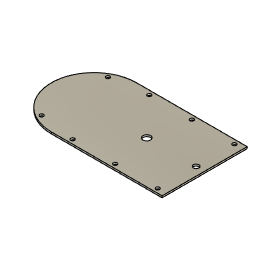
weight_lids v37 (Autodesk Fusion 360 design; units mm, degrees)
Autodesk Fusion 360 part; units mm, degrees
note: some values were not read from the file. Chosen so that the rebuilt part matches the saved one: which face or edge a step refers to; how an offset face is resized. Set by a fixed rule: which sketch regions a step uses.
sketch "Sketch1" plane through (0, 0, 0) normal (0, 0, 1) x (1, 0, 0)
  circle A0 centre (0, 0) radius 45.2465
  dimension "d1" = 90.493
  constraint coincident A0.centre origin
  measures "d1" diameter of A0
sketch "Sketch2" plane through (0, 0, 0) normal (0, 0, 1) x (1, 0, 0)
  circle A0 centre (0, 0) radius 50
  line L0 (0, 0) -> (300, 0)
  line L1 (0, 0) -> (-50, 0)
  circle A1 centre (300, 0) radius 50
  line L2 (300, 0) -> (350, 0)
  line L3 (300, 50) -> (0, 50)
  dimension "d4" = 100
  dimension "d5" = 300
  dimension "d6" = 100
  constraint coincident A0.centre L0.start
  constraint horizontal L0
  constraint coincident A0 L1.end
  constraint parallel L0 L1
  constraint coincident L0.end A1.centre
  constraint coincident A1 L2.end
  constraint parallel L0 L2
  constraint coincident A1 L3.start
  constraint coincident A0 L3.end
  constraint tangent A0 L3
  constraint parallel L0 L3
  measures "d4" diameter of A0
  measures "d5" distance of A0.centre L0.end
  measures "d6" diameter of A1
extrude "Extrude2" add sketch "Sketch2" along normal blind 2 contours A0 L0 L1 | A0 L0 A1 L3 | L0 A1 L2 picked at (-33.1637, 2.3719) picked at (266.8363, 2.3719) makes body 1
sketch "Sketch3" plane through (0, 0, 2) normal (0, 0, 1) x (-1, 0, 0)
  line L0 (50, 0) -> (-350, 0)
  arc A0 (-350, 0) -> (-300, -50) centre (-300, 0) ccw
  line L1 (-300, -50) -> (0, -50)
  arc A1 (0, -50) -> (50, 0) centre (0, 0) ccw
  circle A2 centre (-150, 0) radius 12.7
  dimension "d9" = 25.4
  constraint midpoint L0 A2.centre
  measures "d9" diameter of A2
extrude "Extrude3" cut sketch "Sketch3" against normal blind 30 contours L0 A2 picked at (-150.3164, -4.2215) bodies 1
sketch "Sketch4" plane through (0, 0, 2) normal (0, 0, 1) x (-1, 0, 0)
  arc A0 (-162.7, 0) -> (-137.3, 0) centre (-150, 0) ccw
  line L0 (-162.7, 0) -> (-350, 0)
  arc A1 (-350, 0) -> (-300, -50) centre (-300, 0) ccw
  line L1 (-300, -50) -> (0, -50)
  arc A2 (0, -50) -> (50, 0) centre (0, 0) ccw
  line L2 (50, 0) -> (-137.3, 0)
  circle A3 centre (0, 0) radius 45
  circle A4 centre (-300, 0) radius 45
  line L3 (0, 0) -> (0, -45)
  line L4 (0, -45) -> (-300, -45)
  line L5 (-45, 0) -> (22.5, -38.9711)
  line L6 (22.5, -38.9711) -> (22.5, 38.9711)
  line L7 (22.5, 38.9711) -> (-45, 0)
  line L8 (-255, 0) -> (-322.5, 38.9711)
  line L9 (-322.5, 38.9711) -> (-322.5, -38.9711)
  line L10 (-322.5, -38.9711) -> (-255, 0)
  line L11 (-75, -45) -> (-225, -45)
  line L12 (-225, -45) -> (-225, 0)
  line L13 (-225, 0) -> (-75, 0)
  line L14 (-75, 0) -> (-75, -45)
  line L15 (-175, 0) -> (-125, 0)
  line L16 (-125, 0) -> (-125, -45)
  line L17 (-125, -45) -> (-175, -45)
  line L18 (-175, -45) -> (-175, 0)
  line L19 (-75, 0) -> (-25, 0)
  line L20 (-25, 0) -> (-25, -45)
  line L21 (-25, -45) -> (-75, -45)
  line L22 (-75, -45) -> (-75, 0)
  line L23 (-225, 0) -> (-275, 0)
  line L24 (-275, 0) -> (-275, -45)
  line L25 (-275, -45) -> (-225, -45)
  line L26 (-225, -45) -> (-225, 0)
  point P0 (-300, 0)
  dimension "d12" = 90
  dimension "d13" = 90
  constraint concentric A2 A3
  constraint concentric A1 A4
  constraint coincident A2.centre A3.centre
  constraint coincident A3 L3.end
  constraint perpendicular L2 L3
  constraint coincident A4 L4.end
  constraint tangent A4 L4
  constraint coincident L2 L5.start
  constraint coincident A3 L5.start
  constraint coincident L0 L8.start
  constraint coincident A4 L8.start
  constraint coincident P0 A1.centre
  constraint horizontal L11
  constraint vertical L12
  constraint horizontal L13
  constraint vertical L14
  constraint coincident L0 L12.end
  constraint coincident L4 L11.start
  constraint horizontal L15
  constraint vertical L16
  constraint horizontal L17
  constraint vertical L18
  constraint coincident L4 L16.end
  constraint coincident L13 L15.start
  constraint horizontal L19
  constraint vertical L20
  constraint horizontal L21
  constraint vertical L22
  constraint coincident L4 L20.end
  constraint horizontal L23
  constraint vertical L24
  constraint horizontal L25
  constraint vertical L26
  constraint coincident L4 L24.end
  measures "d12" diameter of A3
  measures "d13" diameter of A4
hole "Hole1" at (-22.5, 38.9711, 2) at (25, 45, 2) at (75, 45, 2) at (125, 45, 2) at (175, 45, 2) at (225, 45, 2) at (275, 45, 2) at (322.5, 38.9711, 2) direction (0, 0, -1) diameter 3.529 depth 70 tip angle 180 bodies 1
thread "Thread1" "ISO Metric profile 4.0 M4x0.5 6H"
sketch "Sketch5" plane through (0, 0, 0) normal (0, 0, 1) x (1, 0, 0)
  circle A0 centre (0, 0) radius 50
  circle A1 centre (300, 0) radius 50
  circle A2 centre (150, 0) radius 12.7
  line L0 (0, -50) -> (300, -50)
  line L1 (50, 0) -> (137.3, 0)
  line L2 (162.7, 0) -> (250, 0)
  line L3 (-50, 0) -> (350, 0)
  dimension "d17" = 25.4
  constraint coincident A0.centre origin
  constraint coincident A0 L0.start
  constraint coincident A1 L0.end
  constraint tangent A1 L0
  constraint horizontal L0
  constraint coincident A0 L1.start
  constraint coincident A2 L1.end
  constraint parallel L0 L1
  constraint coincident A2 L2.start
  constraint coincident A1 L2.end
  constraint parallel L1 L2
  constraint coincident A0 L3.start
  constraint coincident A1 L3.end
  constraint horizontal L3
  measures "d17" diameter of A2
extrude "Extrude4" add sketch "Sketch5" along normal blind 2 contours A0 A1 A2 L0 L1 L2 L3 | A0 L3 | A1 L3 picked at (-6.9236, -15.1605) picked at (285.9791, -9.0107) bodies 1
sketch "Sketch6" plane through (0, 0, 2) normal (0, 0, 1) x (-1, 0, 0)
  circle A0 centre (-150, 0) radius 12.7
  circle A1 centre (-275, -45) radius 1.7644
  circle A2 centre (-175, -45) radius 1.7644
  circle A3 centre (-75, -45) radius 1.7644
  circle A4 centre (22.5, -38.9711) radius 1.7644
  circle A5 centre (-25, -45) radius 1.7644
  circle A6 centre (-125, -45) radius 1.7644
  circle A7 centre (-225, -45) radius 1.7644
  circle A8 centre (-322.5, -38.9711) radius 1.7644
  arc A9 (0, -50) -> (0, 50) centre (0, 0) ccw
  line L0 (0, 50) -> (-300, 50)
  arc A10 (-300, 50) -> (-300, -50) centre (-300, 0) ccw
  line L1 (-300, -50) -> (0, -50)
  line L2 (22.5, -38.9711) -> (22.5, 38.9711)
  line L3 (22.5, 38.9711) -> (-45, 0)
  line L4 (-45, 0) -> (22.5, -38.9711)
  line L5 (-322.5, -38.9711) -> (-255, 0)
  line L6 (-255, 0) -> (-322.5, 38.9711)
  line L7 (-322.5, 38.9711) -> (-322.5, -38.9711)
  line L8 (-25, -45) -> (-25, 50)
  line L9 (-25, 50) -> (-25, 45)
  line L10 (-25, -45) -> (-275, -45)
  line L11 (-275, -45) -> (-275, 45)
  line L12 (-275, 45) -> (-25, 45)
  line L13 (-25, 45) -> (-25, -45)
  line L14 (-25, -45) -> (-75, -45)
  line L15 (-75, -45) -> (-75, 45)
  line L16 (-75, 45) -> (-25, 45)
  line L17 (-25, 45) -> (-25, -45)
  line L18 (-75, -45) -> (-125, -45)
  line L19 (-125, -45) -> (-125, 45)
  line L20 (-125, 45) -> (-75, 45)
  line L21 (-75, 45) -> (-75, -45)
  line L22 (-175, -45) -> (-125, -45)
  line L23 (-125, -45) -> (-125, 45)
  line L24 (-125, 45) -> (-175, 45)
  line L25 (-175, 45) -> (-175, -45)
  line L26 (-225, -45) -> (-175, -45)
  line L27 (-175, -45) -> (-175, 45)
  line L28 (-175, 45) -> (-225, 45)
  line L29 (-225, 45) -> (-225, -45)
  point P0 (-300, 0)
  dimension "d20" = 5
  dimension "d21" = 250
  dimension "d22" = 90
  constraint coincident A4.centre L2.start
  constraint coincident A9.centre origin
  constraint coincident A8.centre L5.start
  constraint coincident P0 A10.centre
  constraint coincident A5.centre L8.start
  constraint coincident L0 L8.end
  constraint perpendicular L0 L8
  constraint perpendicular L0 L9
  constraint horizontal L10
  constraint vertical L11
  constraint horizontal L12
  constraint vertical L13
  constraint horizontal L14
  constraint vertical L15
  constraint horizontal L16
  constraint vertical L17
  constraint coincident L12 L15.end
  constraint horizontal L18
  constraint vertical L19
  constraint horizontal L20
  constraint vertical L21
  constraint coincident L12 L19.end
  constraint horizontal L22
  constraint vertical L23
  constraint horizontal L24
  constraint vertical L25
  constraint coincident A2.centre L22.start
  constraint horizontal L26
  constraint vertical L27
  constraint horizontal L28
  constraint vertical L29
  constraint coincident A7.centre L26.start
  measures "d20" distance of L8.end L9.end
  measures "d21" distance of A5.centre A1.centre
  measures "d22" distance of A5.centre L9.end
hole "Hole2" at (-22.5, -38.9711, 2) at (25, -45, 2) at (75, -45, 2) at (125, -45, 2) at (175, -45, 2) at (225, -45, 2) at (275, -45, 2) at (322.5, -38.9711, 2) direction (0, 0, -1) diameter 3.529 depth 70 tip angle 180 bodies 1
thread "Thread2" "ISO Metric profile 4.0 M4x0.5 6H"
sketch "Sketch7" plane through (0, 0, 2) normal (0, 0, 1) x (-1, 0, 0)
  circle A0 centre (-275, 45) radius 1.7644
  circle A1 centre (-175, 45) radius 1.7644
  circle A2 centre (-75, 45) radius 1.7644
  circle A3 centre (22.5, 38.9711) radius 1.7644
  circle A4 centre (-25, 45) radius 1.7644
  circle A5 centre (-125, 45) radius 1.7644
  circle A6 centre (-225, 45) radius 1.7644
  circle A7 centre (-322.5, 38.9711) radius 1.7644
  circle A8 centre (-150, 0) radius 12.7
  circle A9 centre (-275, -45) radius 1.7644
  circle A10 centre (-175, -45) radius 1.7644
  circle A11 centre (-75, -45) radius 1.7644
  circle A12 centre (22.5, -38.9711) radius 1.7644
  circle A13 centre (-25, -45) radius 1.7644
  circle A14 centre (-125, -45) radius 1.7644
  circle A15 centre (-225, -45) radius 1.7644
  circle A16 centre (-322.5, -38.9711) radius 1.7644
  arc A17 (0, -50) -> (0, 50) centre (0, 0) ccw
  line L0 (0, 50) -> (-300, 50)
  arc A18 (-300, 50) -> (-300, -50) centre (-300, 0) ccw
  line L1 (-300, -50) -> (0, -50)
  line L2 (-150, 0) -> (-130, 0)
  line L3 (-130, 0) -> (-130, -20)
  line L4 (-130, -20) -> (-150, -20)
  line L5 (-150, -20) -> (-150, 0)
  line L6 (-130, -20) -> (-170, -20)
  line L7 (-170, -20) -> (-170, 20)
  line L8 (-170, 20) -> (-130, 20)
  line L9 (-130, 20) -> (-130, -20)
  dimension "d26" = 40
  dimension "d27" = 40
  constraint horizontal L2
  constraint vertical L3
  constraint horizontal L4
  constraint vertical L5
  constraint coincident A8.centre L2.start
  constraint horizontal L6
  constraint vertical L7
  constraint horizontal L8
  constraint vertical L9
  measures "d26" distance of L3.end L6.end
  measures "d27" distance of L3.end L8.end
hole "Hole3" at (130, 20, 2) at (130, -20, 2) at (170, -20, 2) at (170, 20, 2) direction (0, 0, -1) diameter 3.332 depth 70 tip angle 180 bodies 1
ref_plane "WorkPlane1" through (150, 0, 0) normal (1, 0, 0) x (0, 1, 0)
split "Split1" by plane through (150, 0, 0) normal (1, 0, 0) bodies 1 makes body 2 at (206.7848, -6.4118, 0)
sketch "Sketch8" plane through (0, 0, 2) normal (0, 0, 1) x (-1, 0, 0)
  line L0 (-150, -12.7) -> (-150, -50)
  line L1 (-150, -50) -> (0, -50)
  arc A0 (0, -50) -> (0, 50) centre (0, 0) ccw
  line L2 (0, 50) -> (-150, 50)
  line L3 (-150, 50) -> (-150, 12.7)
  arc A1 (-150, -12.7) -> (-150, 12.7) centre (-150, 0) ccw
  circle A2 centre (-130, -20) radius 1.666
  circle A3 centre (-130, 20) radius 1.666
  circle A4 centre (-75, 45) radius 1.7644
  circle A5 centre (22.5, 38.9711) radius 1.7644
  circle A6 centre (-25, 45) radius 1.7644
  circle A7 centre (-125, 45) radius 1.7644
  circle A8 centre (-75, -45) radius 1.7644
  circle A9 centre (22.5, -38.9711) radius 1.7644
  circle A10 centre (-25, -45) radius 1.7644
  circle A11 centre (-125, -45) radius 1.7644
  line L4 (-150, 0) -> (-62, 0)
  line L5 (-150, 0) -> (-238, 0)
  dimension "d32" = 88
  dimension "d33" = 88
  constraint coincident A1.centre L4.start
  constraint parallel L1 L4
  constraint parallel L4 L5
  measures "d32" distance of A1.centre L4.end
  measures "d33" distance of A1.centre L5.end
hole "Hole4" at (62, 0, 2) at (238, 0, 2) direction (0, 0, -1) diameter 6.78 depth 70 tip angle 180 bodies 1 2
thread "Thread4" "ISO Metric profile 8.0 M8x1 6H" major diameter 8.147 minor diameter 7.035 pitch 1 angle 60 resizes the face on face at (62.3375, -3.3732, 1.3333) on face at (238.6717, -3.3228, 1.3333) on bodies 1 2
sketch "Sketch9" plane through (0, 0, 2) normal (0, 0, 1) x (-1, 0, 0)
  circle A0 centre (-62, 0) radius 3.5175
  line L0 (-150, -12.7) -> (-150, -50)
  line L1 (-150, -50) -> (0, -50)
  arc A1 (0, -50) -> (0, 50) centre (0, 0) ccw
  line L2 (0, 50) -> (-150, 50)
  line L3 (-150, 50) -> (-150, 12.7)
  arc A2 (-150, -12.7) -> (-150, 12.7) centre (-150, 0) ccw
  circle A3 centre (-130, -20) radius 1.666
  circle A4 centre (-130, 20) radius 1.666
  circle A5 centre (-75, 45) radius 1.7644
  circle A6 centre (22.5, 38.9711) radius 1.7644
  circle A7 centre (-25, 45) radius 1.7644
  circle A8 centre (-125, 45) radius 1.7644
  circle A9 centre (-75, -45) radius 1.7644
  circle A10 centre (22.5, -38.9711) radius 1.7644
  circle A11 centre (-25, -45) radius 1.7644
  circle A12 centre (-125, -45) radius 1.7644
  circle A13 centre (-150, 0) radius 17.4
  dimension "d37" = 34.8
  constraint concentric A2 A13
  measures "d37" diameter of A13
extrude "Extrude5" cut sketch "Sketch9" against normal blind 10 contours L0 L3 A2 A13 | L0 L3 A2 A13 bodies 1 2
sketch "Sketch10" plane through (0, 0, 2) normal (0, 0, 1) x (-1, 0, 0)
  circle A0 centre (-125, -45) radius 1.7644
  circle A1 centre (-25, -45) radius 1.7644
  circle A2 centre (22.5, -38.9711) radius 1.7644
  circle A3 centre (-75, -45) radius 1.7644
  circle A4 centre (-125, 45) radius 1.7644
  circle A5 centre (-25, 45) radius 1.7644
  circle A6 centre (22.5, 38.9711) radius 1.7644
  circle A7 centre (-75, 45) radius 1.7644
  circle A8 centre (-130, 20) radius 1.666
  circle A9 centre (-130, -20) radius 1.666
  arc A10 (-150, -17.4) -> (-150, 17.4) centre (-150, 0) ccw
  line L0 (-150, -17.4) -> (-150, -50)
  line L1 (-150, -50) -> (0, -50)
  arc A11 (0, -50) -> (0, 50) centre (0, 0) ccw
  line L2 (0, 50) -> (-150, 50)
  line L3 (-150, 50) -> (-150, 17.4)
  circle A12 centre (-62, 0) radius 3.5175
  circle A13 centre (-150, 0) radius 12.7
  circle A14 centre (-150, 0) radius 17.4
  line L4 (-150, -17.4) -> (-150, 17.4)
  dimension "d40" = 25.4
  constraint concentric A10 A13
  constraint concentric A13 A14
  constraint coincident A10.start L0.start
  constraint coincident A10.end L3.end
  measures "d40" diameter of A13
extrude "Extrude6" add sketch "Sketch10" against normal blind 2 contours A10 A13 A14 L4 bodies 1
sketch "Sketch11" plane through (0, 0, 2) normal (0, 0, 1) x (-1, 0, 0)
  circle A0 centre (-170, 20) radius 1.666
  circle A1 centre (-170, -20) radius 1.666
  circle A2 centre (-275, 45) radius 1.7644
  circle A3 centre (-175, 45) radius 1.7644
  circle A4 centre (-225, 45) radius 1.7644
  circle A5 centre (-322.5, 38.9711) radius 1.7644
  arc A6 (-150, 17.4) -> (-150, -17.4) centre (-150, 0) ccw
  line L0 (-150, 17.4) -> (-150, 50)
  line L1 (-150, 50) -> (-300, 50)
  arc A7 (-300, 50) -> (-300, -50) centre (-300, 0) ccw
  line L2 (-300, -50) -> (-150, -50)
  line L3 (-150, -50) -> (-150, -17.4)
  circle A8 centre (-275, -45) radius 1.7644
  circle A9 centre (-175, -45) radius 1.7644
  circle A10 centre (-225, -45) radius 1.7644
  circle A11 centre (-322.5, -38.9711) radius 1.7644
  circle A12 centre (-238, 0) radius 3.5175
  circle A13 centre (-150, 0) radius 12.7
  circle A14 centre (-150, 0) radius 17.4
  line L4 (-150, 17.4) -> (-150, -17.4)
  dimension "d43" = 25.4
  constraint concentric A6 A13
  constraint coincident A6.start L0.start
  constraint coincident A6.end L3.end
  measures "d43" diameter of A13
extrude "Extrude7" add sketch "Sketch11" against normal blind 2 contours A6 A13 A14 L4 bodies 2
sketch "Sketch12" plane through (0, 0, 2) normal (0, 0, 1) x (-1, 0, 0)
  circle A0 centre (-125, -45) radius 1.7644
  circle A1 centre (-25, -45) radius 1.7644
  circle A2 centre (22.5, -38.9711) radius 1.7644
  circle A3 centre (-75, -45) radius 1.7644
  circle A4 centre (-125, 45) radius 1.7644
  circle A5 centre (-25, 45) radius 1.7644
  circle A6 centre (22.5, 38.9711) radius 1.7644
  circle A7 centre (-75, 45) radius 1.7644
  circle A8 centre (-130, 20) radius 1.666
  circle A9 centre (-130, -20) radius 1.666
  line L0 (-150, -12.7) -> (-150, -50)
  line L1 (-150, -50) -> (0, -50)
  arc A10 (0, -50) -> (0, 50) centre (0, 0) ccw
  line L2 (0, 50) -> (-150, 50)
  line L3 (-150, 50) -> (-150, 12.7)
  arc A11 (-150, -12.7) -> (-150, 12.7) centre (-150, 0) ccw
  circle A12 centre (-62, 0) radius 3.5175
  circle A13 centre (-150, 0) radius 20
  dimension "d46" = 40
  constraint concentric A11 A13
  measures "d46" diameter of A13
extrude "Extrude8" cut sketch "Sketch12" against normal blind 2 contours L0 L3 A11 A13 | L0 L3 A11 A13 bodies 1 2
sketch "Sketch13" plane through (0, 0, 2) normal (0, 0, 1) x (-1, 0, 0)
  arc A0 (-150, -20) -> (-150, 20) centre (-150, 0) ccw
  line L0 (-150, -20) -> (-150, -50)
  line L1 (-150, -50) -> (0, -50)
  arc A1 (0, -50) -> (0, 50) centre (0, 0) ccw
  line L2 (0, 50) -> (-150, 50)
  line L3 (-150, 50) -> (-150, 20)
  circle A2 centre (-125, -45) radius 1.7644
  circle A3 centre (-25, -45) radius 1.7644
  circle A4 centre (22.5, -38.9711) radius 1.7644
  circle A5 centre (-75, -45) radius 1.7644
  circle A6 centre (-125, 45) radius 1.7644
  circle A7 centre (-25, 45) radius 1.7644
  circle A8 centre (22.5, 38.9711) radius 1.7644
  circle A9 centre (-75, 45) radius 1.7644
  circle A10 centre (-130, 20) radius 1.666
  circle A11 centre (-130, -20) radius 1.666
  circle A12 centre (-62, 0) radius 3.5175
  line L4 (-150, 0) -> (-122.5, 0)
  line L5 (-150, 0) -> (-177.5, 0)
  dimension "d49" = 27.5
  dimension "d50" = 27.5
  constraint coincident A0.centre L4.start
  constraint parallel L1 L4
  constraint parallel L4 L5
  measures "d49" distance of A0.centre L4.end
  measures "d50" distance of A0.centre L5.end
hole "Hole5" at (122.5, 0, 2) at (177.5, 0, 2) direction (0, 0, -1) diameter 6.78 depth 5 tip angle 180 bodies 1 2
thread "Thread5" "ISO Metric profile 8.0 M8x1 6H" major diameter 8.147 minor diameter 7.035 pitch 1 angle 60 resizes the face on face at (119.7475, 1.9789, 1.3333) on face at (178.1717, -3.3228, 1.3333) on bodies 1 2
extrude "Extrude9" cut 1 faces at (290.9875, -12.4831, 2) along direction (0, 0, -1) blind 2 on bodies 2 bodies 2
delete_face "DeleteFace1" 1 faces at (62.3502, -3.5, 1.3333) on bodies 1
sketch "Sketch14" plane through (0, 0, 2) normal (0, 0, 1) x (-1, 0, 0)
  circle A0 centre (-122.5, 0) radius 3.5175
  arc A1 (-150, -20) -> (-150, 20) centre (-150, 0) ccw
  line L0 (-150, -20) -> (-150, -50)
  line L1 (-150, -50) -> (0, -50)
  arc A2 (0, -50) -> (0, 50) centre (0, 0) ccw
  line L2 (0, 50) -> (-150, 50)
  line L3 (-150, 50) -> (-150, 20)
  circle A3 centre (-125, -45) radius 1.7644
  circle A4 centre (-25, -45) radius 1.7644
  circle A5 centre (22.5, -38.9711) radius 1.7644
  circle A6 centre (-75, -45) radius 1.7644
  circle A7 centre (-125, 45) radius 1.7644
  circle A8 centre (-25, 45) radius 1.7644
  circle A9 centre (22.5, 38.9711) radius 1.7644
  circle A10 centre (-75, 45) radius 1.7644
  circle A11 centre (-130, 20) radius 1.666
  circle A12 centre (-130, -20) radius 1.666
  line L4 (-150, 0) -> (-62, 0)
  circle A13 centre (-62, 0) radius 3.518
  dimension "d56" = 88
  dimension "d57" = 7.036
  constraint coincident A1.centre L4.start
  constraint horizontal L4
  constraint coincident L4.end A13.centre
  measures "d56" distance of A1.centre L4.end
  measures "d57" diameter of A13
extrude "Extrude10" cut sketch "Sketch14" against normal blind 10 contours A13 bodies 1
delete_face "DeleteFace2" 1 faces at (123.8663, 3.2413, 1.3333) on bodies 1
sketch "Sketch15" plane through (0, 0, 2) normal (0, 0, 1) x (-1, 0, 0)
  circle A0 centre (-62, 0) radius 3.518
  arc A1 (-150, -20) -> (-150, 20) centre (-150, 0) ccw
  line L0 (-150, -20) -> (-150, -50)
  line L1 (-150, -50) -> (0, -50)
  arc A2 (0, -50) -> (0, 50) centre (0, 0) ccw
  line L2 (0, 50) -> (-150, 50)
  line L3 (-150, 50) -> (-150, 20)
  circle A3 centre (-125, -45) radius 1.7644
  circle A4 centre (-25, -45) radius 1.7644
  circle A5 centre (22.5, -38.9711) radius 1.7644
  circle A6 centre (-75, -45) radius 1.7644
  circle A7 centre (-125, 45) radius 1.7644
  circle A8 centre (-25, 45) radius 1.7644
  circle A9 centre (22.5, 38.9711) radius 1.7644
  circle A10 centre (-75, 45) radius 1.7644
  circle A11 centre (-130, 20) radius 1.666
  circle A12 centre (-130, -20) radius 1.666
  line L4 (-150, 0) -> (-122.5, 0)
  circle A13 centre (-122.5, 0) radius 3.518
  dimension "d60" = 27.5
  dimension "d61" = 7.036
  constraint coincident A1.centre L4.start
  constraint horizontal L4
  constraint coincident L4.end A13.centre
  measures "d60" distance of A1.centre L4.end
  measures "d61" diameter of A13
extrude "Extrude11" cut sketch "Sketch15" against normal blind 4 contours A13 bodies 1
sketch "Sketch16" plane through (0, 0, 2) normal (0, 0, 1) x (-1, 0, 0)
  circle A0 centre (-122.5, 0) radius 3.518
  circle A1 centre (-62, 0) radius 3.518
  arc A2 (-150, -20) -> (-150, 20) centre (-150, 0) ccw
  line L0 (-150, -20) -> (-150, -50)
  line L1 (-150, -50) -> (0, -50)
  arc A3 (0, -50) -> (0, 50) centre (0, 0) ccw
  line L2 (0, 50) -> (-150, 50)
  line L3 (-150, 50) -> (-150, 20)
  circle A4 centre (-125, -45) radius 1.7644
  circle A5 centre (-25, -45) radius 1.7644
  circle A6 centre (22.5, -38.9711) radius 1.7644
  circle A7 centre (-75, -45) radius 1.7644
  circle A8 centre (-125, 45) radius 1.7644
  circle A9 centre (-25, 45) radius 1.7644
  circle A10 centre (22.5, 38.9711) radius 1.7644
  circle A11 centre (-75, 45) radius 1.7644
  circle A12 centre (-130, 20) radius 1.666
  circle A13 centre (-130, -20) radius 1.666
hole "Hole6" at (-22.5, 38.9711, 2) at (25, 45, 2) at (75, 45, 2) at (125, 45, 2) at (-22.5, -38.9711, 2) at (25, -45, 2) at (75, -45, 2) at (125, -45, 2) direction (0, 0, -1) diameter 4.5 depth 55 tip angle 180 bodies 1
sketch "Sketch17" plane through (0, 0, 2) normal (0, 0, 1) x (-1, 0, 0)
  circle A0 centre (-75, 45) radius 2.25
  circle A1 centre (22.5, 38.9711) radius 2.25
  circle A2 centre (-75, -45) radius 2.25
  circle A3 centre (22.5, -38.9711) radius 2.25
  circle A4 centre (-25, -45) radius 2.25
  circle A5 centre (-125, -45) radius 2.25
  circle A6 centre (-25, 45) radius 2.25
  circle A7 centre (-125, 45) radius 2.25
  circle A8 centre (-122.5, 0) radius 3.518
  circle A9 centre (-62, 0) radius 3.518
  arc A10 (-150, -20) -> (-150, 20) centre (-150, 0) ccw
  line L0 (-150, -20) -> (-150, -50)
  line L1 (-150, -50) -> (0, -50)
  arc A11 (0, -50) -> (0, 50) centre (0, 0) ccw
  line L2 (0, 50) -> (-150, 50)
  line L3 (-150, 50) -> (-150, 20)
  circle A12 centre (-130, 20) radius 1.666
  circle A13 centre (-130, -20) radius 1.666
hole "Hole7" at (130, 20, 2) at (130, -20, 2) direction (0, 0, -1) diameter 4.5 depth 55 tip angle 180 bodies 1
sketch "Sketch18" plane through (0, 0, 2) normal (0, 0, 1) x (-1, 0, 0)
  circle A0 centre (-130, -20) radius 2.25
  circle A1 centre (-130, 20) radius 2.25
  circle A2 centre (-75, 45) radius 2.25
  circle A3 centre (22.5, 38.9711) radius 2.25
  circle A4 centre (-75, -45) radius 2.25
  circle A5 centre (22.5, -38.9711) radius 2.25
  circle A6 centre (-25, -45) radius 2.25
  circle A7 centre (-125, -45) radius 2.25
  circle A8 centre (-25, 45) radius 2.25
  circle A9 centre (-125, 45) radius 2.25
  circle A10 centre (-122.5, 0) radius 3.518
  circle A11 centre (-62, 0) radius 3.518
  arc A12 (-150, -20) -> (-150, 20) centre (-150, 0) ccw
  line L0 (-150, -20) -> (-150, -50)
  line L1 (-150, -50) -> (0, -50)
  arc A13 (0, -50) -> (0, 50) centre (0, 0) ccw
  line L2 (0, 50) -> (-150, 50)
  line L3 (-150, 50) -> (-150, 20)
hole "Hole8" at (62, 0, 2) at (122.5, 0, 2) direction (0, 0, -1) diameter 9 depth 55 tip angle 180 bodies 1
sketch "Sketch19" plane through (0, 0, 2) normal (0, 0, 1) x (-1, 0, 0)
  circle A0 centre (-62, 0) radius 4.5
  circle A1 centre (-122.5, 0) radius 4.5
  circle A2 centre (-130, -20) radius 2.25
  circle A3 centre (-130, 20) radius 2.25
  circle A4 centre (-75, 45) radius 2.25
  circle A5 centre (22.5, 38.9711) radius 2.25
  circle A6 centre (-75, -45) radius 2.25
  circle A7 centre (22.5, -38.9711) radius 2.25
  circle A8 centre (-25, -45) radius 2.25
  circle A9 centre (-125, -45) radius 2.25
  circle A10 centre (-25, 45) radius 2.25
  circle A11 centre (-125, 45) radius 2.25
  arc A12 (-150, -20) -> (-150, 20) centre (-150, 0) ccw
  line L0 (-150, -20) -> (-150, -50)
  line L1 (-150, -50) -> (0, -50)
  arc A13 (0, -50) -> (0, 50) centre (0, 0) ccw
  line L2 (0, 50) -> (-150, 50)
  line L3 (-150, 50) -> (-150, 20)
  circle A14 centre (-150, 0) radius 18
  line L4 (-150, -20) -> (-150, -18)
  line L5 (-150, 20) -> (-150, 18)
  dimension "d73" = 36
  constraint concentric A12 A14
  constraint coincident A12.start L0.start
  constraint coincident A14 L4.end
  constraint parallel L0 L4
  constraint coincident A12.end L3.end
  constraint coincident A14 L5.end
  constraint parallel L3 L5
  measures "d73" diameter of A14
extrude "Extrude12" add sketch "Sketch19" against normal blind 2 contours A12 A14 L4 L5 bodies 1 2
delete_face "DeleteFace3" 1 faces at (131.8901, 21.2207, 1.3333) on bodies 1
delete_face "DeleteFace4" 1 faces at (131.8901, -18.7793, 1.3333) on bodies 1
sketch "Sketch20" plane through (0, 0, 2) normal (0, 0, 1) x (-1, 0, 0)
  circle A0 centre (-62, 0) radius 4.5
  circle A1 centre (-122.5, 0) radius 4.5
  circle A2 centre (-75, 45) radius 2.25
  circle A3 centre (22.5, 38.9711) radius 2.25
  circle A4 centre (-75, -45) radius 2.25
  circle A5 centre (22.5, -38.9711) radius 2.25
  circle A6 centre (-25, -45) radius 2.25
  circle A7 centre (-125, -45) radius 2.25
  circle A8 centre (-25, 45) radius 2.25
  circle A9 centre (-125, 45) radius 2.25
  line L0 (-150, -18) -> (-150, -50)
  line L1 (-150, -50) -> (0, -50)
  arc A10 (0, -50) -> (0, 50) centre (0, 0) ccw
  line L2 (0, 50) -> (-150, 50)
  line L3 (-150, 50) -> (-150, 18)
  arc A11 (-150, -18) -> (-150, 18) centre (-150, 0) ccw
  line L4 (-150, 0) -> (-133.0294, -16.9706)
  line L5 (-133.0294, -16.9706) -> (-150, 0)
  line L6 (-150, 0) -> (-133.0294, 16.9706)
  dimension "d76" = 24
  dimension "d77" = 24
  constraint coincident A11.centre L4.start
  constraint perpendicular L5 L6
  measures "d76" distance of A11.centre L4.end
  measures "d77" distance of A11.centre L6.end
hole "Hole9" at (133.0294, 16.9706, 2) at (133.0294, -16.9706, 2) direction (0, 0, -1) diameter 4.5 depth 10 tip angle 180 bodies 1
delete_face "DeleteFace5" 1 faces at (122.9481, -4.4776, 1.3333) on bodies 1
sketch "Sketch21" plane through (0, 0, 2) normal (0, 0, 1) x (-1, 0, 0)
  circle A0 centre (-133.0294, -16.9706) radius 2.25
  circle A1 centre (-133.0294, 16.9706) radius 2.25
  circle A2 centre (-62, 0) radius 4.5
  circle A3 centre (-75, 45) radius 2.25
  circle A4 centre (22.5, 38.9711) radius 2.25
  circle A5 centre (-75, -45) radius 2.25
  circle A6 centre (22.5, -38.9711) radius 2.25
  circle A7 centre (-25, -45) radius 2.25
  circle A8 centre (-125, -45) radius 2.25
  circle A9 centre (-25, 45) radius 2.25
  circle A10 centre (-125, 45) radius 2.25
  line L0 (-150, -18) -> (-150, -50)
  line L1 (-150, -50) -> (0, -50)
  arc A11 (0, -50) -> (0, 50) centre (0, 0) ccw
  line L2 (0, 50) -> (-150, 50)
  line L3 (-150, 50) -> (-150, 18)
  arc A12 (-150, -18) -> (-150, 18) centre (-150, 0) ccw
  line L4 (-150, 0) -> (-126, 0)
  dimension "d81" = 24
  constraint coincident A12.centre L4.start
  constraint horizontal L4
  measures "d81" distance of A12.centre L4.end
hole "Hole10" at (126, 0, 2) direction (0, 0, -1) diameter 6.6 depth 5 tip angle 180 bodies 1
sketch "Sketch22" plane through (0, 0, 2) normal (0, 0, 1) x (-1, 0, 0)
  circle A0 centre (-126, 0) radius 3.3
  circle A1 centre (-133.0294, -16.9706) radius 2.25
  circle A2 centre (-133.0294, 16.9706) radius 2.25
  circle A3 centre (-62, 0) radius 4.5
  circle A4 centre (-75, 45) radius 2.25
  circle A5 centre (22.5, 38.9711) radius 2.25
  circle A6 centre (-75, -45) radius 2.25
  circle A7 centre (22.5, -38.9711) radius 2.25
  circle A8 centre (-25, -45) radius 2.25
  circle A9 centre (-125, -45) radius 2.25
  circle A10 centre (-25, 45) radius 2.25
  circle A11 centre (-125, 45) radius 2.25
  line L0 (-150, -18) -> (-150, -50)
  line L1 (-150, -50) -> (0, -50)
  arc A12 (0, -50) -> (0, 50) centre (0, 0) ccw
  line L2 (0, 50) -> (-150, 50)
  line L3 (-150, 50) -> (-150, 18)
  arc A13 (-150, -18) -> (-150, 18) centre (-150, 0) ccw
  line L4 (-150, 0) -> (-150, -24)
  line L5 (-150, 0) -> (-150, 24)
  dimension "d85" = 24
  dimension "d86" = 24
  constraint coincident A13.centre L4.start
  constraint vertical L4
  constraint parallel L4 L5
  measures "d85" distance of A13.centre L4.end
  measures "d86" distance of A13.centre L5.end
hole "Hole11" at (150, 24, 2) at (150, -24, 2) direction (0, 0, -1) diameter 6.6 depth 5 tip angle 180 bodies 1
delete_face "DeleteFace6" 1 faces at (126.6539, -3.2346, 1.3333) on bodies 1
delete_face "DeleteFace7" 1 faces at (148.2793, -26.8159, 1.3333) on bodies 1
delete_face "DeleteFace8" 1 faces at (148.2793, 21.1841, 1.3333) on bodies 1
sketch "Sketch23" plane through (0, 0, 2) normal (0, 0, 1) x (-1, 0, 0)
  circle A0 centre (-133.0294, -16.9706) radius 2.25
  circle A1 centre (-133.0294, 16.9706) radius 2.25
  circle A2 centre (-62, 0) radius 4.5
  circle A3 centre (-75, 45) radius 2.25
  circle A4 centre (22.5, 38.9711) radius 2.25
  circle A5 centre (-75, -45) radius 2.25
  circle A6 centre (22.5, -38.9711) radius 2.25
  circle A7 centre (-25, -45) radius 2.25
  circle A8 centre (-125, -45) radius 2.25
  circle A9 centre (-25, 45) radius 2.25
  circle A10 centre (-125, 45) radius 2.25
  line L0 (-150, -18) -> (-150, -50)
  line L1 (-150, -50) -> (0, -50)
  arc A11 (0, -50) -> (0, 50) centre (0, 0) ccw
  line L2 (0, 50) -> (-150, 50)
  line L3 (-150, 50) -> (-150, 18)
  arc A12 (-150, -18) -> (-150, 18) centre (-150, 0) ccw
  circle A13 centre (-150, 0) radius 30
  line L4 (-150, 0) -> (-120, 0)
  line L5 (-150, 0) -> (-150, -30)
  line L6 (-150, 0) -> (-150, 30)
  dimension "d90" = 60
  constraint concentric A12 A13
  constraint coincident A12.centre A13.centre
  constraint coincident A13 L4.end
  constraint horizontal L4
  constraint coincident A13 L5.end
  constraint coincident L0 L5.end
  constraint coincident L3 L6.end
  constraint coincident A13 L6.end
  measures "d90" diameter of A13
hole "Hole12" at (150, 30, 2) at (120, 0, 2) at (150, -30, 2) direction (0, 0, -1) diameter 6.6 depth 10 tip angle 180 bodies 1
delete_face "DeleteFace9" 1 faces at (134.9195, 18.1913, 1.3333) on bodies 1
delete_face "DeleteFace10" 1 faces at (134.9195, -15.7498, 1.3333) on bodies 1
sketch "Sketch24" plane through (0, 0, 2) normal (0, 0, 1) x (-1, 0, 0)
  arc A0 (-150, -33.3) -> (-150, -26.7) centre (-150, -30) ccw
  line L0 (-150, -33.3) -> (-150, -50)
  line L1 (-150, -50) -> (0, -50)
  arc A1 (0, -50) -> (0, 50) centre (0, 0) ccw
  line L2 (0, 50) -> (-150, 50)
  line L3 (-150, 50) -> (-150, 33.3)
  arc A2 (-150, 26.7) -> (-150, 33.3) centre (-150, 30) ccw
  line L4 (-150, 26.7) -> (-150, 18)
  arc A3 (-150, -18) -> (-150, 18) centre (-150, 0) ccw
  line L5 (-150, -18) -> (-150, -26.7)
  circle A4 centre (-125, 45) radius 2.25
  circle A5 centre (-25, 45) radius 2.25
  circle A6 centre (-125, -45) radius 2.25
  circle A7 centre (-25, -45) radius 2.25
  circle A8 centre (22.5, -38.9711) radius 2.25
  circle A9 centre (-75, -45) radius 2.25
  circle A10 centre (22.5, 38.9711) radius 2.25
  circle A11 centre (-75, 45) radius 2.25
  circle A12 centre (-62, 0) radius 4.5
  circle A13 centre (-120, 0) radius 3.3
  circle A14 centre (-150, 0) radius 30
  line L6 (-150, 0) -> (-128.7868, -21.2132)
  line L7 (-150, 0) -> (-120, 0) construction
  line L8 (-150, 0) -> (-128.7868, 21.2132)
  dimension "d94" = 60
  dimension "d95" = 30
  dimension "d96" = 45
  dimension "d97" = 30
  constraint concentric A3 A14
  constraint horizontal L7
  constraint coincident A3.centre A14.centre
  constraint perpendicular L6 L8
  measures "d94" diameter of A14
  measures "d95" distance of A3.centre L6.end
  measures "d96" angle of L6 L7
  measures "d97" distance of A3.centre L8.end
hole "Hole13" at (128.7868, 21.2132, 2) at (128.7868, -21.2132, 2) direction (0, 0, -1) diameter 4.5 depth 10 tip angle 180 bodies 1
sketch "Sketch25" plane through (0, 0, 2) normal (0, 0, 1) x (-1, 0, 0)
  circle A0 centre (-128.7868, -21.2132) radius 2.25
  circle A1 centre (-128.7868, 21.2132) radius 2.25
  arc A2 (-150, -33.3) -> (-150, -26.7) centre (-150, -30) ccw
  line L0 (-150, -33.3) -> (-150, -50)
  line L1 (-150, -50) -> (0, -50)
  arc A3 (0, -50) -> (0, 50) centre (0, 0) ccw
  line L2 (0, 50) -> (-150, 50)
  line L3 (-150, 50) -> (-150, 33.3)
  arc A4 (-150, 26.7) -> (-150, 33.3) centre (-150, 30) ccw
  line L4 (-150, 26.7) -> (-150, 18)
  arc A5 (-150, -18) -> (-150, 18) centre (-150, 0) ccw
  line L5 (-150, -18) -> (-150, -26.7)
  circle A6 centre (-125, 45) radius 2.25
  circle A7 centre (-25, 45) radius 2.25
  circle A8 centre (-125, -45) radius 2.25
  circle A9 centre (-25, -45) radius 2.25
  circle A10 centre (22.5, -38.9711) radius 2.25
  circle A11 centre (-75, -45) radius 2.25
  circle A12 centre (22.5, 38.9711) radius 2.25
  circle A13 centre (-75, 45) radius 2.25
  circle A14 centre (-62, 0) radius 4.5
  circle A15 centre (-120, 0) radius 3.3
  circle A16 centre (-150, 0) radius 25
  dimension "d101" = 50
  constraint concentric A5 A16
  measures "d101" diameter of A16
extrude "Extrude13" cut sketch "Sketch25" against normal blind 10 contours L4 A5 L5 A16 picked at (-127.4349, 1.6343) bodies 1
sketch "Sketch26" plane through (0, 0, 2) normal (0, 0, 1) x (-1, 0, 0)
  arc A0 (-150, -25) -> (-150, 25) centre (-150, 0) ccw
  line L0 (-150, -25) -> (-150, -26.7)
  arc A1 (-150, -33.3) -> (-150, -26.7) centre (-150, -30) ccw
  line L1 (-150, -33.3) -> (-150, -50)
  line L2 (-150, -50) -> (0, -50)
  arc A2 (0, -50) -> (0, 50) centre (0, 0) ccw
  line L3 (0, 50) -> (-150, 50)
  line L4 (-150, 50) -> (-150, 33.3)
  arc A3 (-150, 26.7) -> (-150, 33.3) centre (-150, 30) ccw
  line L5 (-150, 26.7) -> (-150, 25)
  circle A4 centre (-128.7868, -21.2132) radius 2.25
  circle A5 centre (-128.7868, 21.2132) radius 2.25
  circle A6 centre (-125, 45) radius 2.25
  circle A7 centre (-25, 45) radius 2.25
  circle A8 centre (-125, -45) radius 2.25
  circle A9 centre (-25, -45) radius 2.25
  circle A10 centre (22.5, -38.9711) radius 2.25
  circle A11 centre (-75, -45) radius 2.25
  circle A12 centre (22.5, 38.9711) radius 2.25
  circle A13 centre (-75, 45) radius 2.25
  circle A14 centre (-62, 0) radius 4.5
  circle A15 centre (-120, 0) radius 3.3
  circle A16 centre (-150, 0) radius 35
  dimension "d104" = 70
  constraint concentric A0 A16
  measures "d104" diameter of A16
extrude "Extrude14" cut sketch "Sketch26" against normal blind 10 contours A0 L0 A1 L1 L4 A3 L5 A16 picked at (-143.1599, -29.075) bodies 1
sketch "Sketch27" plane through (0, 0, 2) normal (0, 0, 1) x (-1, 0, 0)
  circle A0 centre (-62, 0) radius 4.5
  circle A1 centre (-75, 45) radius 2.25
  circle A2 centre (22.5, 38.9711) radius 2.25
  circle A3 centre (-75, -45) radius 2.25
  circle A4 centre (22.5, -38.9711) radius 2.25
  circle A5 centre (-25, -45) radius 2.25
  circle A6 centre (-125, -45) radius 2.25
  circle A7 centre (-25, 45) radius 2.25
  circle A8 centre (-125, 45) radius 2.25
  arc A9 (-150, -35) -> (-150, 35) centre (-150, 0) ccw
  line L0 (-150, -35) -> (-150, -50)
  line L1 (-150, -50) -> (0, -50)
  arc A10 (0, -50) -> (0, 50) centre (0, 0) ccw
  line L2 (0, 50) -> (-150, 50)
  line L3 (-150, 50) -> (-150, 35)
  line L4 (-150, -35) -> (-115, -35)
  line L5 (-115, -35) -> (-115, 35)
  line L6 (-115, 35) -> (-150, 35)
  line L7 (-150, 35) -> (-150, -35)
  dimension "d107" = 35
  dimension "d108" = 70
  constraint horizontal L4
  constraint vertical L5
  constraint horizontal L6
  constraint vertical L7
  constraint coincident A9.start L0.start
  measures "d107" distance of A9.start L4.end
  measures "d108" distance of A9.start A9.end
extrude "Extrude15" cut sketch "Sketch27" against normal blind 5 contours A9 L4 L5 | A9 L5 L6 bodies 1
sketch "Sketch28" plane through (0, 0, 2) normal (0, 0, 1) x (-1, 0, 0)
  line L0 (-115, -35) -> (-150, -35)
  line L1 (-150, -35) -> (-150, -50)
  line L2 (-150, -50) -> (0, -50)
  arc A0 (0, -50) -> (0, 50) centre (0, 0) ccw
  line L3 (0, 50) -> (-150, 50)
  line L4 (-150, 50) -> (-150, 35)
  line L5 (-150, 35) -> (-115, 35)
  line L6 (-115, 35) -> (-115, -35)
  circle A1 centre (-62, 0) radius 4.5
  circle A2 centre (-75, 45) radius 2.25
  circle A3 centre (22.5, 38.9711) radius 2.25
  circle A4 centre (-75, -45) radius 2.25
  circle A5 centre (22.5, -38.9711) radius 2.25
  circle A6 centre (-25, -45) radius 2.25
  circle A7 centre (-125, -45) radius 2.25
  circle A8 centre (-25, 45) radius 2.25
  circle A9 centre (-125, 45) radius 2.25
  line L7 (-115, -35) -> (-135, -35)
  line L8 (-135, -35) -> (-135, -15)
  line L9 (-135, -15) -> (-115, -15)
  line L10 (-115, -15) -> (-115, -35)
  line L11 (-115, 35) -> (-135, 35)
  line L12 (-135, 35) -> (-135, 15)
  line L13 (-135, 15) -> (-115, 15)
  line L14 (-115, 15) -> (-115, 35)
  dimension "d111" = 20
  dimension "d112" = 20
  dimension "d113" = 20
  dimension "d114" = 20
  constraint horizontal L7
  constraint vertical L8
  constraint horizontal L9
  constraint vertical L10
  constraint coincident L0.start L6.end
  constraint horizontal L11
  constraint vertical L12
  constraint horizontal L13
  constraint vertical L14
  constraint coincident L5.end L6.start
  measures "d111" distance of L0.start L7.end
  measures "d112" distance of L0.start L9.end
  measures "d113" distance of L5.end L11.end
  measures "d114" distance of L5.end L13.end
extrude "Extrude16" add sketch "Sketch28" against normal blind 2 contours L0 L6 L7 L8 L9 L10 | L5 L6 L11 L12 L13 L14 bodies 1
sketch "Sketch29" plane through (0, 0, 2) normal (0, 0, 1) x (-1, 0, 0)
  line L0 (-135, -35) -> (-150, -35)
  line L1 (-150, -35) -> (-150, -50)
  line L2 (-150, -50) -> (0, -50)
  arc A0 (0, -50) -> (0, 50) centre (0, 0) ccw
  line L3 (0, 50) -> (-150, 50)
  line L4 (-150, 50) -> (-150, 35)
  line L5 (-150, 35) -> (-135, 35)
  line L6 (-135, 35) -> (-135, 15)
  line L7 (-135, 15) -> (-115, 15)
  line L8 (-115, 15) -> (-115, -15)
  line L9 (-115, -15) -> (-135, -15)
  line L10 (-135, -15) -> (-135, -35)
  circle A1 centre (-62, 0) radius 4.5
  circle A2 centre (-75, 45) radius 2.25
  circle A3 centre (22.5, 38.9711) radius 2.25
  circle A4 centre (-75, -45) radius 2.25
  circle A5 centre (22.5, -38.9711) radius 2.25
  circle A6 centre (-25, -45) radius 2.25
  circle A7 centre (-125, -45) radius 2.25
  circle A8 centre (-25, 45) radius 2.25
  circle A9 centre (-125, 45) radius 2.25
  line L11 (-150, 0) -> (-128.7868, -21.2132)
  line L12 (-150, 0) -> (-120, 0) construction
  line L13 (-150, 0) -> (-128.7868, 21.2132)
  line L14 (-150, 0) -> (-120, 0) construction
  dimension "d118" = 30
  dimension "d119" = 45
  dimension "d120" = 45
  dimension "d121" = 30
  constraint horizontal L12
  constraint horizontal L14
  measures "d118" distance of L11.start L11.end
  measures "d119" angle of L11 L12
  measures "d120" angle of L13 L14
  measures "d121" distance of L11.start L13.end
hole "Hole14" at (128.7868, 21.2132, 2) at (128.7868, -21.2132, 2) direction (0, 0, -1) diameter 4.5 depth 10 tip angle 180 bodies 1
extrude "Extrude17" cut 2 faces at (150, 45, 1.3333) (150, -45, 1.3333) along direction (-1, 0, 0) blind 15 on bodies 1 bodies 1
extrude "Extrude18" cut 1 faces at (115, 5, 1.3333) along direction (-1, 0, 0) blind 5 on bodies 1 bodies 1
extrude "Extrude19" add 1 faces at (110, 5, 1.3333) along direction (1, 0, 0) blind 25 on bodies 1 bodies 1
delete_face "DeleteFace11" 1 faces at (130.6769, 22.4339, 1.3333) on bodies 1
delete_face "DeleteFace12" 1 faces at (130.6769, -19.9925, 1.3333) on bodies 1
sketch "Sketch30" plane through (0, 0, 2) normal (0, 0, 1) x (-1, 0, 0)
  line L0 (-135, 50) -> (-135, -50)
  line L1 (-135, -50) -> (0, -50)
  arc A0 (0, -50) -> (0, 50) centre (0, 0) ccw
  line L2 (0, 50) -> (-135, 50)
  circle A1 centre (-62, 0) radius 4.5
  circle A2 centre (-75, 45) radius 2.25
  circle A3 centre (22.5, 38.9711) radius 2.25
  circle A4 centre (-75, -45) radius 2.25
  circle A5 centre (22.5, -38.9711) radius 2.25
  circle A6 centre (-25, -45) radius 2.25
  circle A7 centre (-125, -45) radius 2.25
  circle A8 centre (-25, 45) radius 2.25
  circle A9 centre (-125, 45) radius 2.25
  line L3 (-135, 0) -> (-120, 0)
  dimension "d131" = 15
  constraint midpoint L0 L3.start
  constraint perpendicular L0 L3
  measures "d131" distance of L3.start L3.end
hole "Hole15" at (120, 0, 2) direction (0, 0, -1) diameter 6.6 depth 20 tip angle 180 bodies 1
extrude "Extrude20" cut 1 faces at (135, 16.6667, 0.6667) along direction (-1, 0, 0) blind 5 on bodies 1 bodies 1
delete_face "DeleteFace13" 1 faces at (125.874, -42.9267, 1.3333) on bodies 1
delete_face "DeleteFace14" 1 faces at (125.874, 47.0733, 1.3333) on bodies 1
delete_face "DeleteFace15" 1 faces at (75.874, -42.9267, 1.3333) on bodies 1
delete_face "DeleteFace16" 1 faces at (75.874, 47.0733, 1.3333) on bodies 1
sketch "Sketch31" plane through (0, 0, 2) normal (0, 0, 1) x (-1, 0, 0)
  line L0 (-130, 50) -> (-130, -50)
  line L1 (-130, -50) -> (0, -50)
  arc A0 (0, -50) -> (0, 50) centre (0, 0) ccw
  line L2 (0, 50) -> (-130, 50)
  circle A1 centre (-120, 0) radius 3.3
  circle A2 centre (-62, 0) radius 4.5
  circle A3 centre (22.5, 38.9711) radius 2.25
  circle A4 centre (22.5, -38.9711) radius 2.25
  circle A5 centre (-25, -45) radius 2.25
  circle A6 centre (-25, 45) radius 2.25
  line L3 (-25, 45) -> (-20, 45)
  line L4 (-20, 45) -> (-70, 45)
  line L5 (-70, 45) -> (-120, 45)
  line L6 (-25, -45) -> (-20, -45)
  line L7 (-20, -45) -> (-70, -45)
  line L8 (-70, -45) -> (-71.8524, -45)
  line L9 (-71.8524, -45) -> (-121.8524, -45)
  dimension "d137" = 5
  dimension "d138" = 50
  dimension "d139" = 50
  dimension "d140" = 5
  dimension "d141" = 50
  dimension "d142" = 50
  constraint coincident A6.centre L3.start
  constraint horizontal L3
  constraint parallel L3 L4
  constraint horizontal L5
  constraint coincident A5.centre L6.start
  constraint horizontal L6
  constraint parallel L6 L7
  constraint horizontal L8
  constraint parallel L8 L9
  measures "d137" distance of A6.centre L3.end
  measures "d138" distance of L3.end L4.end
  measures "d139" distance of L4.end L5.end
  measures "d140" distance of A5.centre L6.end
  measures "d141" distance of L6.end L7.end
  measures "d142" distance of L8.end L9.end
delete_face "DeleteFace17" 1 faces at (22.8672, -45.7166, 1.3333) on bodies 1
delete_face "DeleteFace18" 1 faces at (22.8672, 44.2834, 1.3333) on bodies 1
hole "Hole16" at (20, 45, 2) at (20, -45, 2) at (70, -45, 2) at (70, 45, 2) at (121.8524, 45, 2) at (120, -45, 2) direction (0, 0, -1) diameter 4.5 depth 20 tip angle 180 bodies 1
sketch "Sketch32" plane through (0, 0, 2) normal (0, 0, 1) x (-1, 0, 0)
  circle A0 centre (-121.8524, -45) radius 2.25
  circle A1 centre (-70, 45) radius 2.25
  circle A2 centre (-20, -45) radius 2.25
  circle A3 centre (-20, 45) radius 2.25
  circle A4 centre (-70, -45) radius 2.25
  circle A5 centre (-120, 45) radius 2.25
  line L0 (-130, 50) -> (-130, -50)
  line L1 (-130, -50) -> (0, -50)
  arc A6 (0, -50) -> (0, 50) centre (0, 0) ccw
  line L2 (0, 50) -> (-130, 50)
  circle A7 centre (-120, 0) radius 3.3
  circle A8 centre (-62, 0) radius 4.5
  circle A9 centre (22.5, 38.9711) radius 2.25
  circle A10 centre (22.5, -38.9711) radius 2.25
  line L3 (-70, -45) -> (-120, -45)
  dimension "d146" = 50
  constraint coincident A4.centre L3.start
  constraint horizontal L3
  measures "d146" distance of A4.centre L3.end
delete_face "DeleteFace19" 1 faces at (122.7264, 47.0733, 1.3333) on bodies 1
hole "Hole17" at (120, 45, 2) direction (0, 0, -1) diameter 4.5 depth 10 tip angle 180 bodies 1
equation "d40 = ( 12.7 * 2 ) * 1 mm"
equation "d43 = ( 12.7 * 2 ) * 1 mm"
equation "d57 = ( 3.518 * 2 ) * 1 mm"
equation "d61 = ( 3.518 * 2 ) * 1 mm"
